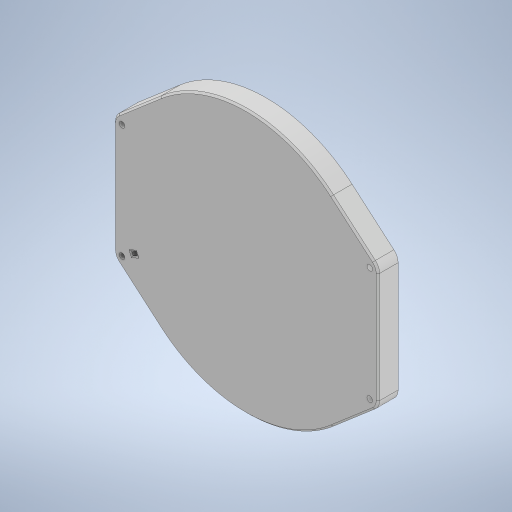
# Autodesk Inventor part: Body
Saved by Autodesk Inventor 2024 (Build 280153000, 153)
## iProperties
Created: 2024-01-24
Part Number: Body
Material: Generic
Document SubType Name: Modeling
Designer: crow
Density: 1 g/cm^3
Appearance: Default
Mass: 314.708 g
Surface Area: 1457.7 cm^2
Volume: 314.708 cm^3
Author: crow
Autodesk Inventor part; units mm, degrees
ref_plane "YZ Plane" through (0, 0, 0) normal (1, 0, 0) x (0, 1, 0)
ref_plane "XZ Plane" through (0, 0, 0) normal (0, 1, 0) x (-1, 0, 0)
sketch "Sketch1" plane through (0, 0, 0) normal (0, 0, 1) x (1, 0, 0)
  line L0 (95.8, -44.0209) -> (95.8, 44.0209)
  line L1 (95.8, 44.0209) -> (0, 126.2524)
  circle A0 centre (0, 0) radius 90.9
  line L2 (-95.8, 44.0209) -> (-95.8, -44.0209)
  line L3 (0, -126.2524) -> (95.8, -44.0209)
  line L4 (0, 126.2524) -> (-95.8, 44.0209)
  line L5 (-95.8, -44.0209) -> (0, -126.2524)
  dimension "d47" = 181.8
  constraints: 12 end point, 4 equal length, 4 vertical, 1 centre point, 4 other
  measures "d47" diameter of A0
extrude "Extrusion3" add sketch "Sketch1" along normal blind 14.65
ref_plane "Work Plane1" through (0, 0, 8.9) normal (0, 0, 1) x (1, 0, 0)
sketch "Sketch2" plane through (0, 0, 8.9) normal (0, 0, 1) x (1, 0, 0)
  circle A0 centre (0, 0) radius 90.9 projected
  circle A1 centre (0, 0) radius 86.6
  circle A2 centre (0, 0) radius 90.9 projected
  line L0 (95.8, -44.0209) -> (95.8, 44.0209) projected
  line L1 (0, -126.2524) -> (95.8, -44.0209) projected
  line L2 (-95.8, -44.0209) -> (0, -126.2524) projected
  line L3 (-95.8, 44.0209) -> (-95.8, -44.0209) projected
  line L4 (0, 126.2524) -> (-95.8, 44.0209) projected
  line L5 (95.8, 44.0209) -> (0, 126.2524) projected
  dimension "d54" = 4.3
  constraints: 1 centre point, 1 coincident
  measures "d54" radial gap between concentric circles of A0 A1
extrude "Extrusion2" add sketch "Sketch2" along normal blind 5.75 contours A1
sketch "Sketch3" plane through (0, 0, 14.65) normal (0, 0, 1) x (1, 0, 0)
  line L0 (-78.7096, -36.1158) -> (-82.6168, -37.9113)
  circle A0 centre (0, 0) radius 89 projected
  circle A1 centre (0, 0) radius 89 projected
  circle A2 centre (0, 0) radius 90.9 projected
  circle A3 centre (0, 0) radius 90.9 projected
  line L1 (95.8, -44.0209) -> (0, -126.2524) projected
  line L2 (0, -126.2524) -> (-95.8, -44.0209) projected
  line L3 (-95.8, -44.0209) -> (-95.8, 44.0209) projected
  line L4 (-95.8, 44.0209) -> (0, 126.2524) projected
  line L5 (0, 126.2524) -> (95.8, 44.0209) projected
  line L6 (95.8, 44.0209) -> (95.8, -44.0209) projected
  circle A4 centre (0, 0) radius 90.9 projected
  line L7 (95.8, -44.0209) -> (95.8, 44.0209) projected
  line L8 (0, -126.2524) -> (95.8, -44.0209) projected
  line L9 (-95.8, -44.0209) -> (0, -126.2524) projected
  line L10 (-95.8, 44.0209) -> (-95.8, -44.0209) projected
  line L11 (0, 126.2524) -> (-95.8, 44.0209) projected
  line L12 (95.8, 44.0209) -> (0, 126.2524) projected
  circle A5 centre (0, 0) radius 86.6 projected
  circle A6 centre (0, 0) radius 86.6 projected
  line L13 (-83.8258, -35.1575) -> (-79.8629, -33.4885)
  point P0 (-84.0051, -35.376)
  point P1 (-80.4353, -36.9088)
  point P2 (-83.8258, -35.1575)
  dimension "d55" = 2.93
  constraints: 4 end point, 4 point on circle, 1 point on line, 1 other
  measures "d55" distance from line of L13 point (-80.435, -36.909)
extrude "Extrusion1" add sketch "Sketch3" against normal blind 2.5 contours A5 L13 A0 L0 | A0 L13 A2 L0 picked at (24.8672, -83.6168) picked at (89.616, 8.8098)
fillet "Fillet9" radius 0.8 1 edges at (-81.8443, -34.323, 12.15)
fillet "Fillet8" radius 0.8 1 edges at (-80.6632, -37.0136, 12.15)
fillet "Fillet7" radius 0.8 2 edges at (-80.6632, -37.0136, 14.65) (-83.2327, -36.5394, 14.65)
fillet "Fillet7" radius 0.8 2 edges at (-79.2971, -34.8069, 14.65) (-81.8443, -34.323, 14.65)
fillet "Fillet6" radius 8.7504 1 edges at (-95.8, 44.0209, 7.325)
fillet "Fillet5" radius 8.7504 1 edges at (-95.8, -44.0209, 7.325)
fillet "Fillet4" radius 8.7504 1 edges at (95.8, 44.0209, 7.325)
fillet "Fillet3" radius 8.7504 1 edges at (95.8, -44.0209, 7.325)
fillet "Fillet2" radius 95.8 1 edges at (0, -126.2524, 7.325)
fillet "Fillet1" radius 95.8 1 edges at (0, 126.2524, 7.325)
chamfer "Chamfer1" distance 1.25 angle 45 12 edges at (0, -95.8, 14.65) (-95.0007, 43.6536, 14.65) (77.573, -59.6663, 14.65) (-77.573, 59.6663, 14.65) (95.0007, -43.6536, 14.65) (0, 95.8, 14.65) (77.573, 59.6663, 14.65) (-95.0007, -43.6536, 14.65) (95.0007, 43.6536, 14.65) (-95.8, 0, 14.65) (-77.573, -59.6663, 14.65) (95.8, 0, 14.65)
hole "Hole4" at (-89.8894, 41.3049, 14.65) direction (0, 0, -1) diameter 4 depth 14.65 tip angle 118
hole "Hole3" at (89.8894, -41.3049, 14.65) direction (0, 0, -1) diameter 4 depth 14.65 tip angle 118
sketch "Sketch5" plane through (0, 0, 14.65) normal (0, 0, 1) x (1, 0, 0)
  point P0 (89.8894, -41.3049)
hole "Hole2" at (-89.8894, -41.3049, 14.65) direction (0, 0, -1) diameter 4 depth 14.65 tip angle 118
sketch "Sketch4" plane through (0, 0, 14.65) normal (0, 0, 1) x (1, 0, 0)
  point P0 (-89.8894, 41.3049)
hole "Hole1" at (89.8894, 41.3049, 14.65) direction (0, 0, -1) diameter 4 depth 14.65 tip angle 118
sketch "Sketch8" plane through (0, 0, 0) normal (1, 0, 0) x (0, 1, 0)
  line L0 (-91, 1) -> (-93.3, 1)
  line L1 (-88, 1.25) -> (-90, 1.25)
  line L2 (-93.3, 1) -> (-93.3, 0)
  line L3 (-90, 4.25) -> (-91, 4.25)
  line L4 (-90, 4.25) -> (-90, 1.25)
  line L5 (-88, 0) -> (-93.3, 0)
  line L6 (-91, 4.25) -> (-91, 1)
  line L7 (-88, 1.25) -> (-88, 0)
  line L8 (0, 0) -> (0, -10)
  constraints: 18 end point, 5 vertical, 4 horizontal, 1 perpendicular
revolve "Revolution1" [suppressed]
sketch "Sketch9" plane through (0, 0, 0) normal (1, 0, 0) x (0, 1, 0)
  line L0 (-91, 1) -> (-93.3, 1)
  line L1 (-93.3, 1) -> (-93.3, 0)
  line L2 (0, 0) -> (-93.3, 0)
  line L3 (-91, 4.25) -> (-91, 1)
  line L4 (0, 4.25) -> (-91, 4.25)
  line L5 (0, 0) -> (0, 4.25)
  line L6 (0, 0) -> (0, -10)
  constraints: 14 end point, 4 vertical, 3 horizontal
revolve "Revolution2" [suppressed]
sketch "Sketch10" plane through (0, 0, 0) normal (1, 0, 0) x (0, 1, 0)
  line L0 (0, 4.25) -> (90, 4.25)
  line L1 (90, 4.25) -> (90, 1.25)
  line L2 (90, 1.25) -> (88, 1.25)
  line L3 (88, 1.25) -> (88, 0)
  line L4 (88, 0) -> (0, 0)
  line L5 (0, 0) -> (0, 4.25)
  line L6 (0, 4.25) -> (0, 0)
  constraints: 14 end point, 3 horizontal, 3 vertical, 1 collinear
revolve "Revolution3" [suppressed]
sketch "Sketch6" plane through (0, 0, 14.65) normal (0, 0, 1) x (1, 0, 0)
  point P0 (-89.8894, -41.3049)
sketch "Sketch7" plane through (0, 0, 14.65) normal (0, 0, 1) x (1, 0, 0)
  point P0 (89.8894, 41.3049)
body "Solid3"
body "Solid4"
body "Solid5"
